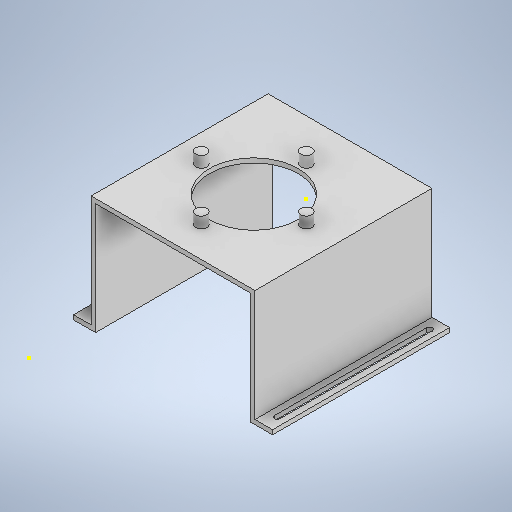
# Autodesk Inventor part: caja
Saved by Autodesk Inventor 2025.2 (Build 292293000, 293)
## iProperties
Created: 2026-09-20
Part Number: caja
Material: Generic
Document SubType Name: Sheet Metal
Designer: dguar
Density: 1 g/cm^3
Sheet Metal Rule: Default_mm
Appearance: Default
Author: dguar
Autodesk Inventor part; units mm, degrees
ref_plane "YZ Plane" through (0, 0, 0) normal (1, 0, 0) x (0, 1, 0)
ref_plane "XZ Plane" through (0, 0, 0) normal (0, 1, 0) x (-1, 0, 0)
ref_plane "XY Plane" through (0, 0, 0) normal (0, 0, 1) x (1, 0, 0)
sketch "Sketch1" plane through (0, 0, 0) normal (0, 1, 0) x (-1, 0, 0)
  point P0 (0, 0)
sketch "Sketch2" plane through (0, 0, 0) normal (0, 0, 1) x (1, 0, 0)
  line L0 (0, 0) -> (0, 4)
  line L1 (160, 0) -> (160, 4)
  line L2 (0, 0) -> (9.95, 0)
  line L3 (160, 0) -> (150.05, 0)
  line L4 (150.05, 0) -> (150.05, 101)
  line L5 (150.05, 101) -> (9.95, 101)
  line L6 (9.95, 101) -> (9.95, 0)
  line L7 (0, 4) -> (5.95, 4)
  line L8 (5.95, 4) -> (5.95, 101)
  line L9 (5.95, 101) -> (5.95, 105)
  line L10 (5.95, 105) -> (150.05, 105)
  line L11 (150.05, 105) -> (154.05, 105)
  line L12 (154.05, 105) -> (154.05, 4)
  line L13 (154.05, 4) -> (160, 4)
  line L14 (0, 0) -> (9.95, 0)
  line L15 (150.05, 0) -> (160, 0)
  constraints: 32 end point, 5 perpendicular, 3 vertical, 2 horizontal, 2 point on line, 1 parallel
extrude "Extrusion1" add sketch "Sketch2" along normal blind 250
sketch "Sketch3" plane through (5.95, 105, 0) normal (0, 1, 0) x (1, 0, 0)
  line L0 (0, 0) -> (0, -250) projected
  line L1 (144.1, 0) -> (144.1, -250) projected
  circle A0 centre (72.05, -125) radius 40
  point P0 (-5.95, 0)
  dimension "d15" = 80
  constraints: 1 centre point
  measures "d15" diameter of A0
extrude "Extrusion2" cut sketch "Sketch3" against normal blind 250
sketch "Sketch4" plane through (0, 0, 250) normal (0, 0, 1) x (1, 0, 0)
  point P0 (0, 0)
sketch "Sketch5" plane through (0, 0, 250) normal (0, 0, 1) x (1, 0, 0)
  line L0 (0, 0) -> (165.9252, 0)
  line L1 (165.9252, 0) -> (165.9252, 113.7831)
  line L2 (165.9252, 113.7831) -> (0, 113.7831)
  line L3 (0, 113.7831) -> (0, 0)
  constraints: 8 end point, 2 parallel, 1 horizontal, 1 perpendicular
extrude "Extrusion3" cut sketch "Sketch5" against normal blind 50
sketch "Sketch6" plane through (0, 0, 0) normal (0, 0, -1) x (-1, 0, 0)
  line L0 (0, 4) -> (0, 0) projected
  line L1 (0, 0) -> (-198.2615, 0)
  line L2 (-198.2615, 0) -> (-198.2615, 123.0797)
  line L3 (-198.2615, 123.0797) -> (0, 123.0797)
  line L4 (0, 123.0797) -> (0, 0)
  constraints: 8 end point, 2 parallel, 1 horizontal, 1 perpendicular
extrude "Extrusion4" cut sketch "Sketch6" against normal blind 40
sketch "Sketch7" plane through (160, 0, 200) normal (1, 0, 0) x (0, 0, -1)
  line L0 (0, 0) -> (0, 4) projected
  line L1 (160, 0) -> (0, 0) projected
  line L2 (0, 4) -> (160, 4)
  line L3 (160, 4) -> (160, 0)
  line L4 (160, 0) -> (0, 0)
  line L5 (0, 0) -> (0, 4)
  point P0 (200, 0)
  constraints: 8 end point, 2 parallel, 1 horizontal, 1 perpendicular
extrude "Extrusion5" add sketch "Sketch7" along normal blind 10
sketch "Sketch8" plane through (0, 0, 200) normal (-1, 0, 0) x (0, 0, 1)
  line L0 (-160, 0) -> (0, 0) projected
  line L1 (-160, 4) -> (0, 4)
  line L2 (0, 4) -> (0, 0)
  line L3 (0, 0) -> (-160, 0)
  line L4 (-160, 0) -> (-160, 4)
  point P0 (-200, 0)
  constraints: 8 end point, 2 parallel, 1 horizontal, 1 perpendicular
extrude "Extrusion6" add sketch "Sketch8" along normal blind 10
sketch "Sketch9" plane through (5.95, 4, 200) normal (0, 1, 0) x (1, 0, 0)
  line L0 (0, 160) -> (0, 0) projected
  line L1 (0, 0) -> (-15.95, 0) projected
  arc A0 (-5.475, 149.5645) -> (-10.475, 149.5645) centre (-7.975, 149.5645) ccw
  arc A1 (-10.475, 11.8823) -> (-5.475, 11.8823) centre (-7.975, 11.8823) ccw
  line L2 (-10.475, 11.8823) -> (-10.475, 149.5645)
  line L3 (-5.475, 11.8823) -> (-5.475, 149.5645)
  line L4 (164.05, 0) -> (164.05, 160) projected
  line L5 (164.05, 0) -> (148.5752, 0)
  line L6 (164.05, 0) -> (144.1, 0) projected
  line L7 (144.1, 160) -> (164.05, 160) projected
  arc A2 (153.8126, 11.8823) -> (158.8126, 11.8823) centre (156.3126, 11.8823) ccw
  arc A3 (158.8126, 149.5645) -> (153.8126, 149.5645) centre (156.3126, 149.5645) ccw
  line L8 (153.8126, 11.8823) -> (153.8126, 149.5645)
  line L9 (158.8126, 11.8823) -> (158.8126, 149.5645)
  point P0 (-5.95, 200)
  point P1 (-15.95, 160)
  dimension "d26" = 5
  dimension "d27" = 5
  dimension "d28" = 5
  dimension "d29" = 5
  constraints: 10 end point, 8 point on circle, 4 centre point, 4 tangent, 1 parallel, 1 point on line
  measures "d26" diameter of A0
  measures "d27" diameter of A1
  measures "d28" diameter of A2
  measures "d29" diameter of A3
extrude "Extrusion7" cut sketch "Sketch9" against normal blind 10
sketch "Sketch10" plane through (5.95, 105, 200) normal (0, 1, 0) x (1, 0, 0)
  circle A0 centre (72.05, 75) radius 40 projected
  line L0 (0, 0) -> (148.1, 0) projected
  line L1 (4, 160) -> (4, 0) projected
  line L2 (144.1, 160) -> (144.1, 0) projected
  circle A1 centre (119.55, 75) radius 5
  circle A2 centre (72.05, 27.5) radius 5
  circle A3 centre (24.55, 75) radius 5
  circle A4 centre (72.05, 122.5) radius 5
  point P0 (-5.95, 200)
  dimension "d35" = 10
  dimension "d39" = 10
  dimension "d40" = 10
  dimension "d41" = 10
  constraints: 4 centre point
  measures "d35" diameter of A1
  measures "d39" diameter of A2
  measures "d40" diameter of A3
  measures "d41" diameter of A4
extrude "Extrusion8" add sketch "Sketch10" along normal blind 10 contours A1 | A2 | A3 | A4
equation "\"BendRadius\" = Thickness"
equation "\"BendReliefWidth\" = Thickness"
equation "\"BendReliefDepth\" = 0.5 * Thickness"
equation "\"CornerReliefSize\" = 4 * Thickness"
equation "\"MinimumRemnant\" = 2 * Thickness"
equation "\"TransitionRadius\" = BendRadius"
equation "\"JacobiRadiusSize\" = BendRadius"
equation "\"GapSize\" = Thickness"
equation "\"Thickness\" = 0.5"
body "Solid1"
